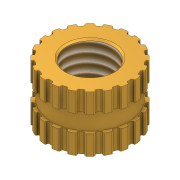
# Autodesk Inventor part: Insert Brass M5
Saved by Autodesk Inventor 2021 (Build 250183000, 183)
## iProperties
Created: 2021-12-09
Part Number: Insert Brass M5
Material: Brass, Soft Yellow
Document SubType Name: Modeling
Designer: MSI Bravo
Density: 8.47 g/cm^3
Appearance: Brass - Satin
Author: MSI Bravo
Autodesk Inventor part; units mm, degrees
ref_plane "YZ Plane" through (0, 0, 0) normal (1, 0, 0) x (0, 1, 0)
ref_plane "XZ Plane" through (0, 0, 0) normal (0, 1, 0) x (-1, 0, 0)
ref_plane "XY Plane" through (0, 0, 0) normal (0, 0, 1) x (1, 0, 0)
sketch "Sketch1" plane through (0, 0, 0) normal (0, 1, 0) x (-1, 0, 0)
  circle A0 centre (0, 0) radius 3.75
  dimension "d0" = 7.5
  constraints: 1 centre point, 1 coincident
  measures "d0" diameter of A0
extrude "Extrusion1" add sketch "Sketch1" along normal mid plane 5
sketch "Sketch2" plane through (0, 0, 0) normal (0, 1, 0) x (-1, 0, 0)
  circle A0 centre (0, 0) radius 3.75 projected
  circle A1 centre (0, 0) radius 3.45
  dimension "d3" = 6.9
  constraints: 1 centre point
  measures "d3" diameter of A1
extrude "Extrusion2" cut sketch "Sketch2" along normal mid plane 1.5
sketch "Sketch3" plane through (0, 2.5, 0) normal (0, 1, 0) x (1, 0, 0)
  circle A0 centre (0, 0) radius 3.75 projected
  constraints: 1 coincident
hole "Hole1" at (0, 2.5, 0) direction (0, -1, 0) diameter 4.134 depth 14.2 tip angle 118 thread size "M5x0.8" class "6H" standard "ISO Metric profile"
sketch "Sketch4" plane through (0, 2.5, 0) normal (0, 1, 0) x (1, 0, 0)
  circle A0 centre (0, 0) radius 3.75 projected
  circle A1 centre (0, 0) radius 3.5
  line L0 (-0.25, 4.1331) -> (0.25, 4.1331)
  line L1 (0.25, 4.1331) -> (0.25, 2.7925)
  line L2 (0.25, 2.7925) -> (-0.25, 2.7925)
  line L3 (-0.25, 2.7925) -> (-0.25, 4.1331)
  point P0 (0, 4.1331)
  point P1 (-0.25, 3.7417)
  point P2 (-0.25, 3.4911)
  point P3 (0.25, 3.4911)
  point P4 (0.25, 3.7417)
  dimension "d13" = 7
  dimension "d14" = 0.5
  constraints: 8 end point, 2 parallel, 1 centre point, 1 horizontal, 1 midpoint, 1 perpendicular, 1 vertical alignment
  measures "d13" diameter of A1
  measures "d14" distance of L0.start L0.end
extrude "Extrusion3" cut sketch "Sketch4" against normal through all contours L1 A1 L3 A0 picked at (0.1945, 3.5772)
pattern_circular "Circular Pattern1" count 20 over 360 about axis through (0, -4.6, 0) along (0, 1, 0) of "Extrusion3"
chamfer "Chamfer1" distance 0.15 angle 45 2 edges at (0, 2.5, -2.067) (0, -2.5, -2.067)
fillet "Fillet1" radius 0.1 8 edges at (-3.6358, 1.625, -0.9185) (-3.7417, 1.625, -0.25) (-3.3974, 1.625, -0.841) (-3.4911, 1.625, -0.25) (-3.3974, -1.625, -0.841) (-3.4911, -1.625, -0.25) (-3.7417, -1.625, -0.25) (-3.6358, -1.625, -0.9185)
pattern_circular "Circular Pattern2" count 20 over 360 about axis through (0, -4.6, 0) along (0, 1, 0) of "Fillet1"
body "Solid1"
